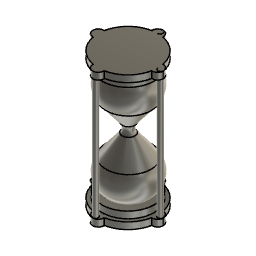
sandglass (Autodesk Fusion 360 design; units mm, degrees)
Autodesk Fusion 360 part; units mm, degrees
sketch "Sketch28" plane through (0, 0, 0) normal (0, 1, 0) x (1, 0, 0)
sketch "Sketch29" plane through (0, 0, 0) normal (0, 1, 0) x (1, 0, 0)
sketch "Sketch30" plane through (0, 0, 0) normal (0, 1, 0) x (-1, 0, 0)
sketch "Sketch31" plane through (0, 0, 0) normal (0, 1, 0) x (1, 0, 0)
sketch "Sketch32" plane through (0, 0, 0) normal (0, 1, 0) x (1, 0, 0)
sketch "Sketch33" plane through (0, 0, 0) normal (0, 1, 0) x (1, 0, 0)
sketch "Sketch34" plane through (0, 0, 0) normal (0, 1, 0) x (1, 0, 0)
sketch "Sketch35" plane through (0, 0, 0) normal (0, 1, 0) x (-1, 0, 0)
  line L0 (74.525367, 81.716092) -> (75.805367, 81.716092)
  line L1 (76.225367, 97.416092) -> (74.525367, 97.416092)
  line L2 (80.571265, 88.545162) -> (76.22504, 82.941884)
  arc A0 (80.571265, 88.545162) -> (76.225367, 97.416092) centre (76.225367, 91.916092) ccw
  arc A1 (76.22504, 82.941884) -> (75.805367, 81.716092) centre (77.805367, 81.716092) ccw
  line L3 (76.225367, 66.016092) -> (74.525367, 66.016092)
  arc A2 (76.225367, 66.016092) -> (80.571265, 74.887021) centre (76.225367, 71.516092) ccw
  line L4 (80.571265, 74.887021) -> (76.22504, 80.490299)
  arc A3 (75.805367, 81.716092) -> (76.22504, 80.490299) centre (77.805367, 81.716092) ccw
  line L5 (76.225367, 96.416092) -> (74.525367, 96.416092)
  arc A4 (79.781102, 89.158058) -> (76.225367, 96.416092) centre (76.225367, 91.916092) ccw
  line L6 (79.781102, 89.158058) -> (75.434877, 83.55478)
  arc A5 (75.434877, 83.55478) -> (74.805367, 81.716092) centre (77.805367, 81.716092) ccw
  arc A6 (74.805367, 81.716092) -> (75.434877, 79.877403) centre (77.805367, 81.716092) ccw
  line L7 (79.781102, 74.274125) -> (75.434877, 79.877403)
  arc A7 (76.225367, 67.016092) -> (79.781102, 74.274125) centre (76.225367, 71.516092) ccw
  line L8 (76.225367, 67.016092) -> (74.525367, 67.016092)
  line L9 (74.525367, 66.016092) -> (74.525367, 67.016092)
  line L10 (74.525367, 96.416092) -> (74.525367, 97.416092)
  dimension "d52" = 4
  dimension "d54" = 3.28
  dimension "d55" = 1.7
  dimension "d58" = 1
  constraint vertical L9
  constraint perpendicular L1 L9
  constraint tangent L2 A1
  constraint symmetric L0 A0 A2
  constraint symmetric L0 A1 A3
  constraint collinear L9 L10
  measures "d52" diameter of A1
revolve "Revolve1" add sketch "Sketch35" angle 360 about axis through (-74.525367, 0, 96.416092) along (0, 0, 1) contours L0 L1 L2 A0 A1 L5 A4 L6 A5 L10 | L0 L3 A2 L4 A3 A6 L7 A7 L8 L9 picked at (77.410394, 85.013942) picked at (77.147006, 78.213942) makes body 1
move_body "Move1" bodies 1 to x (1, 0, 0) y (0, 1, 0) z (0, 0, 1) at (60, 30, 0)
move_body "Move2" bodies 1 to x (1, 0, 0) y (0, 1, 0) z (0, 0, 1) at (22.06817, -36.579772, -58.647941)
move_body "Move3" bodies 1 to x (1, 0, 0) y (0, 1, 0) z (0, 0, 1) at (-7, 7, 0)
sketch "Sketch36" plane through (0, 0, 0) normal (0, 0, 1) x (1, 0, 0)
  circle A0 centre (0, 0) radius 8
  circle A1 centre (0, 8) radius 1.5
  circle A2 centre (8, 0) radius 1.5
  circle A3 centre (0, -8) radius 1.5
  circle A4 centre (-8, 0) radius 1.5
  circle A5 centre (8.7, -0.000674) radius 0.7
  circle A6 centre (0.000674, 8.699832) radius 0.699832
  circle A7 centre (-8.7, 0) radius 0.7
  circle A8 centre (0, -8.7) radius 0.7
  constraint coincident A0.centre origin
  constraint coincident A0 A1.centre
  constraint coincident A0 A2.centre
  constraint coincident A0 A3.centre
  constraint coincident A0 A4.centre
  constraint coincident A4.centre A7
  constraint tangent A0 A7
  constraint coincident A3.centre A8
  constraint tangent A0 A8
  constraint tangent A0 A6
  constraint tangent A0 A5
extrude "Extrude8" add sketch "Sketch36" along normal blind 1.8 separate body contours A0 A2 | A0 A2 | A0 A1 A2 A3 A4 | A0 A1 | A0 A1 | A0 A3 | A0 A3 | A0 A4 | A0 A4 picked at (7.516433, -0.312355) picked at (8.285716, 1.02424) picked at (0, 2.166667) picked at (-0.312011, 7.516441) picked at (1.035599, 8.291632) picked at (1.03536, -8.291684) picked at (-0.312355, -7.516433) picked at (-7.516433, -0.312355) picked at (-8.294141, -1.02147) makes body 2
sketch "Sketch37" plane through (0, 0, 1.8) normal (0, 0, 1) x (-1, 0, 0)
  circle A0 centre (-8.7, 0.000674) radius 0.7
  circle A1 centre (0, 8.7) radius 0.7
  circle A2 centre (-0.000674, -8.699832) radius 0.699832
  circle A3 centre (8.7, 0) radius 0.7
  arc A4 (1.493393, -7.859375) -> (7.859375, -1.493393) centre (0, 0) ccw
  arc A5 (7.859375, -1.493393) -> (7.859375, 1.493393) centre (8, 0) ccw
  arc A6 (7.859375, 1.493393) -> (1.493393, 7.859375) centre (0, 0) ccw
  arc A7 (1.493393, 7.859375) -> (-1.493393, 7.859375) centre (0, 8) ccw
  arc A8 (-1.493393, 7.859375) -> (-7.859375, 1.493394) centre (0, 0) ccw
  arc A9 (-7.859375, 1.493394) -> (-7.859375, -1.493394) centre (-8, 0) ccw
  arc A10 (-7.859375, -1.493394) -> (-1.493393, -7.859375) centre (0, 0) ccw
  arc A11 (-1.493393, -7.859375) -> (1.493393, -7.859375) centre (0, -8) ccw
  circle A12 centre (0, 0) radius 7
  constraint concentric A4 A12
extrude "Extrude9" add sketch "Sketch37" along normal blind 1.8 contours A12 picked at (-1.45481, -1.128743) bodies 2
move_body "Move4" bodies 1 to x (1, 0, 0) y (0, 1, 0) z (0, 0, 1) at (-1.029961, -0.782957, -4.898832)
move_body "Move5" bodies 1 to x (1, 0, 0) y (0, 1, 0) z (0, 0, 1) at (0.5, 0.5, 0)
ref_plane "WorkPlane1" through (0, 0, 18) normal (0, 0, 1) x (1, 0, 0)
mirror "Mirror1" about plane through (0, 0, 18) normal (0, 0, 1) of "Extrude8", "Extrude9" makes body 3
sketch "Sketch38" plane through (0, 0, 0) normal (1, 0, 0) x (0, 1, 0)
sketch "Sketch39" plane through (0, 0, 0) normal (0, 0, 1) x (1, 0, 0)
  circle A0 centre (8.7, 0) radius 0.7
  circle A1 centre (0, 8.7) radius 0.7
  circle A2 centre (-8.7, 0) radius 0.7
  circle A3 centre (0, -8.7) radius 0.7
extrude "Extrude10" cut sketch "Sketch39" along normal blind 36 contours A0 | A1 | A2 | A3 picked at (8.956844, -0.217204) picked at (0.171045, 8.858707) picked at (-8.443155, -0.217204) picked at (0.171045, -8.541293) bodies 2 3
sketch "Sketch40" plane through (0, 0, 18) normal (0, 0, 1) x (1, 0, 0)
  circle A0 centre (0, 8.7) radius 0.7
  circle A1 centre (-8.7, 0) radius 0.7
  circle A2 centre (0, -8.7) radius 0.7
  circle A3 centre (8.7, 0) radius 0.7
extrude "Extrude11" add sketch "Sketch40" along normal mid plane 36 contours A0 | A1 | A2 | A3 picked at (0.171045, 8.858707) picked at (-8.443155, -0.217204) picked at (0.171045, -8.541293) picked at (8.956844, -0.217204) bodies 2 3
